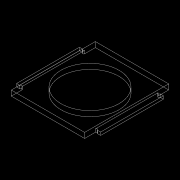
# Autodesk Inventor part: JointA2
Saved by Autodesk Inventor 2011 (Build 150239000, 239)
## iProperties
Created: 2012-10-15
Part Number: JointA2
Document SubType Name: Modeling
Designer: JohnHenry
Density: 1 g/cm^3
Author: JohnHenry
Autodesk Inventor part; units mm, degrees
ref_plane "YZ Plane" through (0, 0, 0) normal (1, 0, 0) x (0, 1, 0)
ref_plane "XZ Plane" through (0, 0, 0) normal (0, 1, 0) x (-1, 0, 0)
ref_plane "XY Plane" through (0, 0, 0) normal (0, 0, 1) x (1, 0, 0)
sketch "スケッチ1" plane through (0, 0, 0) normal (0, 0, 1) x (1, 0, 0)
  circle A0 centre (0, 0) radius 27.6
  line L0 (-40, 40) -> (40, 40)
  line L1 (40, 40) -> (40, -40)
  line L2 (40, -40) -> (-40, -40)
  line L3 (-40, -40) -> (-40, 40)
  dimension "d0" = 55.2
  dimension "d1" = 40
  dimension "d2" = 80
  dimension "d3" = 80
  dimension "d4" = 40
  constraints: 8 end point, 2 parallel, 1 centre point, 1 coincident, 1 horizontal, 1 perpendicular
  measures "d0" diameter of A0
  measures "d1" distance from line of L0 A0.centre
  measures "d2" distance of L0.end L1.end
  measures "d3" distance of L0.start L0.end
  measures "d4" distance from line of L1 point (0, 0)
extrude "押し出し1" add sketch "スケッチ1" along normal blind 5
sketch "スケッチ3" plane through (0, 0, 5) normal (0, 0, 1) x (1, 0, 0)
  line L0 (40, -40) -> (-40, -40) projected
  line L1 (-40, 40) -> (-34.9, 40)
  line L2 (-34.9, 40) -> (-34.9, -40)
  line L3 (-34.9, -40) -> (-40, -40)
  line L4 (-40, -40) -> (-40, 40)
  line L5 (40, 40) -> (34.9, 40)
  line L6 (34.9, 40) -> (34.9, -40)
  line L7 (34.9, -40) -> (40, -40)
  line L8 (40, -40) -> (40, 40)
  dimension "d17" = 5.1
  dimension "d18" = 5.1
  constraints: 16 end point, 4 parallel, 2 horizontal, 2 perpendicular, 2 point on line
  measures "d17" distance of L2.end L3.end
  measures "d18" distance between parallel lines of L8 L6
extrude "押し出し3" cut sketch "スケッチ3" against normal blind 2.2
sketch "スケッチ4" plane through (0, 0, 0) normal (0, 0, -1) x (-1, 0, 0)
  line L0 (-40, 40) -> (-34.9, 40)
  line L1 (-34.9, 40) -> (-34.9, 29.9)
  line L2 (-34.9, 29.9) -> (-40, 29.9)
  line L3 (-40, 29.9) -> (-40, 40)
  line L4 (-40, -40) -> (-34.9, -40)
  line L5 (-34.9, -40) -> (-34.9, -29.9)
  line L6 (-34.9, -29.9) -> (-40, -29.9)
  line L7 (-40, -29.9) -> (-40, -40)
  line L8 (40, 40) -> (34.9, 40)
  line L9 (34.9, 40) -> (34.9, 29.9)
  line L10 (34.9, 29.9) -> (40, 29.9)
  line L11 (40, 29.9) -> (40, 40)
  line L12 (40, -40) -> (34.9, -40)
  line L13 (34.9, -40) -> (34.9, -29.9)
  line L14 (34.9, -29.9) -> (40, -29.9)
  line L15 (40, -29.9) -> (40, -40)
  dimension "d21" = 5.1
  dimension "d22" = 10.1
  dimension "d23" = 10.1
  dimension "d24" = 10.1
  dimension "d25" = 5.1
  dimension "d26" = 5.1
  dimension "d27" = 5.1
  dimension "d28" = 10.1
  constraints: 32 end point, 8 parallel, 4 horizontal, 4 perpendicular
  measures "d21" distance of L1.end L2.end
  measures "d22" distance of L0.end L1.end
  measures "d23" distance of L4.end L5.end
  measures "d24" distance of L10.end L8.start
  measures "d25" distance of L9.end L10.end
  measures "d26" distance of L5.end L6.end
  measures "d27" distance of L13.end L14.end
  measures "d28" distance of L12.end L13.end
extrude "押し出し4" cut sketch "スケッチ4" against normal through all
sketch "スケッチ5" plane through (0, 0, 0) normal (0, 0, -1) x (-1, 0, 0)
  line L0 (-40, -29.9) -> (-34.9, -29.9) projected
  line L1 (-34.9, -29.9) -> (-34.9, -40) projected
  line L2 (34.9, -40) -> (34.9, -29.9) projected
  line L3 (34.9, -29.9) -> (40, -29.9) projected
  line L4 (40, 29.9) -> (34.9, 29.9) projected
  line L5 (34.9, 29.9) -> (34.9, 40) projected
  line L6 (-34.9, 40) -> (-34.9, 29.9) projected
  line L7 (-34.9, 29.9) -> (-40, 29.9) projected
  point P0 (-35.9, 29.9)
  point P1 (-35.9, -29.9)
  point P2 (35.9, -29.9)
  point P3 (35.9, 29.9)
  dimension "d31" = 1
  dimension "d32" = 1
  dimension "d33" = 1
  dimension "d34" = 1
  constraints: 4 point on line
  measures "d31" distance from line of L6 point (-35.9, 29.9)
  measures "d32" distance from line of L1 point (-35.9, -29.9)
  measures "d33" distance from line of L5 point (35.9, 29.9)
  measures "d34" distance from line of L2 point (35.9, -29.9)
hole "Hole1" at (35.9, 29.9, 0) at (35.9, -29.9, 0) at (-35.9, -29.9, 0) at (-35.9, 29.9, 0) direction (0, 0, 1) diameter 2 end through all
equation "\"d1\" = 0.5 * d2"
equation "\"d3\" = d2"
equation "\"d4\" = d1"
equation "\"d18\" = d17"
equation "\"d23\" = d22"
equation "\"d25\" = d21"
equation "\"d26\" = d21"
equation "\"d27\" = d21"
equation "\"d28\" = d22"
equation "\"d32\" = d31"
equation "\"d33\" = d31"
equation "\"d34\" = d31"
